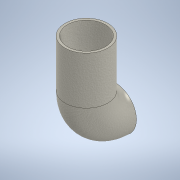
# Autodesk Inventor part: Intake
Saved by Autodesk Inventor 2021 (Build 250183000, 183)
## iProperties
Created: 2021-04-23
Part Number: Intake
Material: Stainless Steel
Document SubType Name: Modeling
Designer: lucia
Density: 8 g/cm^3
Appearance: Steel - Cast
Author: lucia
Autodesk Inventor part; units mm, degrees
ref_plane "YZ Plane" through (0, 0, 0) normal (1, 0, 0) x (0, 1, 0)
ref_plane "XZ Plane" through (0, 0, 0) normal (0, 1, 0) x (-1, 0, 0)
ref_plane "XY Plane" through (0, 0, 0) normal (0, 0, 1) x (1, 0, 0)
sketch "Sketch1" plane through (0, 0, 0) normal (0, 0, 1) x (1, 0, 0)
  circle A0 centre (0, 0) radius 12.7
  circle A1 centre (0, 0) radius 14.2875
  dimension "d0" = 28.575
  dimension "d1" = 25.4
  constraints: 2 centre point, 2 coincident
  measures "d0" diameter of A1
  measures "d1" diameter of A0
sketch "Sketch2" plane through (0, 0, 0) normal (1, 0, 0) x (0, 1, 0)
  arc A0 (19.05, 19.05) -> (0, 0) centre (19.05, 0) ccw
  dimension "d2" = 19.05
  dimension "d3" = 19.05
  constraints: 2 point on circle, 1 centre point
  measures "d2" radius of A0
  measures "d3" horizontal distance of A0.end A0.start
sweep "Sweep1" add profiles "Sketch1" path "Sketch2"
sketch "Sketch3" plane through (0, 19.05, 19.05) normal (0, 1, 0) x (1, 0, 0)
  circle A0 centre (0, 0) radius 12.7
  circle A1 centre (0, 0) radius 14.2875
  point P0 (0, 19.05)
  dimension "d6" = 25.4
  dimension "d7" = 28.575
  dimension "d8" = 19.05
  constraints: 2 centre point, 1 coincident
  measures "d6" diameter of A0
  measures "d7" diameter of A1
  measures "d8" distance of point (0, 19.05) A0.centre
extrude "Extrusion1" add sketch "Sketch3" along normal blind 31.75
body "Solid1"
